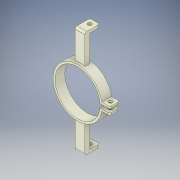
# Autodesk Inventor part: SupportBracket_BilgePumpMotor
Saved by Autodesk Inventor 2019 (Build 230136000, 136)
## iProperties
Created: 2019-03-02
Part Number: SupportBracket_BilgePumpMotor
Material: ABS Plastic
Document SubType Name: Modeling
Designer: User
Density: 1.06 g/cm^3
Appearance: Smooth - Ivory
Author: User
Autodesk Inventor part; units mm, degrees
ref_plane "XY Plane" through (0, 0, 0) normal (0, 0, 1) x (1, 0, 0)
sketch "Sketch1" plane through (0, 0, 0) normal (0, 0, 1) x (1, 0, 0)
  arc A0 (22.9129, 2) -> (22.9129, -2) centre (0, 0) ccw
  arc A1 (24.6779, 4) -> (24.6779, -4) centre (0, 0) ccw
  line L0 (22.9129, 2) -> (24.9199, 2)
  line L1 (22.9129, -2) -> (24.9199, -2)
  line L2 (24.9199, 2) -> (32.9199, 2)
  line L3 (32.9199, 2) -> (32.9199, 4)
  line L4 (32.9199, 4) -> (24.6779, 4)
  line L5 (24.9199, -2) -> (32.9199, -2)
  line L6 (32.9199, -2) -> (32.9199, -4)
  line L7 (32.9199, -4) -> (24.6779, -4)
  dimension "d0" = 46
  dimension "d1" = 50
  dimension "d7" = 2
  dimension "d9" = 2
  constraints: 16 end point, 4 point on circle, 2 centre point, 2 coincident, 2 horizontal, 2 parallel, 2 perpendicular
  measures "d0" diameter of A0
  measures "d1" diameter of A1
  measures "d7" distance of L3.end L2.end
  measures "d9" distance of L5.end L6.end
extrude "Extrusion1" add sketch "Sketch1" against normal blind 10
sketch "Sketch2" plane through (24.6779, 4, 0) normal (0, 1, 0) x (1, 0, 0)
  line L0 (8.2419, 0) -> (0, 0) projected
  line L1 (8.2419, 0) -> (8.2419, 10) projected
  line L2 (0, 10) -> (8.2419, 10) projected
  line L3 (0, 0) -> (0, 10) projected
  circle A0 centre (4.121, 5) radius 2
  point P0 (-24.6779, 0)
  dimension "d12" = 4
  constraints: 1 centre point
  measures "d12" diameter of A0
extrude "Extrusion2" cut sketch "Sketch2" against normal blind 8.5 contours A0
ref_plane "Work Plane1" through (24.6779, 24, 0) normal (0, 1, 0) x (1, 0, 0)
sketch "Sketch3" plane through (24.6779, 24, 0) normal (0, 1, 0) x (1, 0, 0)
  line L0 (-24.6779, 0) -> (-24.6779, 10)
  line L1 (-19.6779, 7.5) -> (-29.6779, 7.5)
  line L2 (-29.6779, 2.5) -> (-19.6779, 2.5)
  line L3 (-19.6779, 2.5) -> (-19.6779, 7.5)
  line L4 (-29.6779, 2.5) -> (-29.6779, 7.5)
  point P0 (-24.6779, 5)
  constraints: 10 end point, 1 coincident, 1 midpoint, 1 parallel, 1 vertical
extrude "Extrusion3" add sketch "Sketch3" along normal blind 27.5
sketch "Sketch4" plane through (5, 24.4949, -6) normal (1, 0, 0) x (0, 0, -1)
  line L0 (1.5, 27.0051) -> (-3.5, 27.0051) projected
  line L1 (-3.5, 27.0051) -> (11.5, 27.0051)
  line L2 (11.5, 27.0051) -> (11.5, 30.0051)
  line L3 (11.5, 30.0051) -> (-3.5, 30.0051)
  line L4 (-3.5, 30.0051) -> (-3.5, 27.0051)
  point P0 (-6, -24.4949)
  dimension "d27" = 15
  dimension "d28" = 3
  constraints: 8 end point, 2 parallel, 1 horizontal, 1 perpendicular
  measures "d27" distance of L3.end L2.end
  measures "d28" distance of L2.end L1.end
extrude "Extrusion4" add sketch "Sketch4" against normal blind 10
ref_plane "Work Plane2" through (0, 0, 0) normal (0.7071, -0.7071, 0) x (0, 0, -1)
sketch "Sketch5" plane through (5, 54.5, -2.5) normal (0, 1, 0) x (1, 0, 0)
  circle A0 centre (-5, 10) radius 2
  dimension "d29" = 4
  constraints: 1 centre point
  measures "d29" diameter of A0
extrude "Extrusion5" cut sketch "Sketch5" against normal blind 4
mirror "Mirror2" about plane through (0, 0, 0) normal (0, 1, 0) of "Extrusion4", "Extrusion5", "Extrusion3"
fillet "Fillet1" radius 2 10 edges at (0, 54.5, -2.5) (5, 53, -17.5) (-5, 53, -17.5) (5, -53, -17.5) (-5, -53, -17.5) (0, -54.5, -2.5) (32.9199, 3, 0) (32.9199, 3, -10) (32.9199, -3, 0) (32.9199, -3, -10)
body "Solid1"
